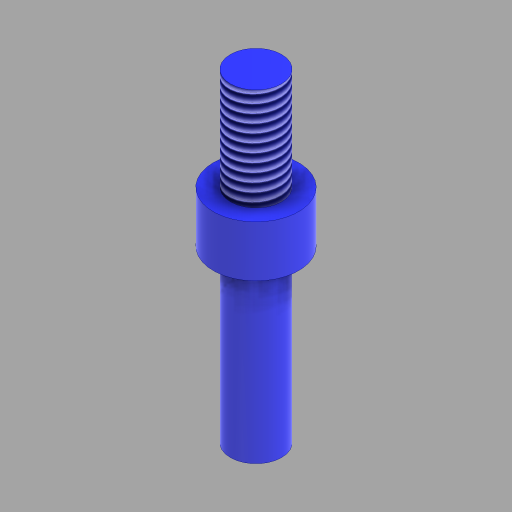
# Autodesk Inventor part: Fitting-1
Saved by Autodesk Inventor 2024 (Build 280153020, 153B)
## iProperties
Created: 2023-09-24
Part Number: Fitting-1
Material: Brass
Document SubType Name: Modeling
Designer: schanen
Density: 8.49 g/cm^3
Appearance: Blue - Wall Paint - Glossy
Author: schanen
Autodesk Inventor part; units mm, degrees
ref_plane "YZ Plane" through (0, 0, 0) normal (1, 0, 0) x (0, 1, 0)
ref_plane "XZ Plane" through (0, 0, 0) normal (0, 1, 0) x (-1, 0, 0)
ref_plane "XY Plane" through (0, 0, 0) normal (0, 0, 1) x (1, 0, 0)
sketch "Sketch1" plane through (0, 0, 0) normal (0, 0, 1) x (1, 0, 0)
  line L0 (0, 19) -> (-1.5, 19)
  line L1 (-1.5, 19) -> (-1.5, 13)
  line L2 (-1.5, 13) -> (-2.5, 13)
  line L3 (-2.5, 13) -> (-2.5, 10)
  line L4 (-2.5, 10) -> (-1.5, 10)
  line L5 (-1.5, 10) -> (-1.5, 0)
  line L6 (-1.5, 0) -> (0, 0)
  line L7 (0, 0) -> (0, 19)
  dimension "d0" = 1.5
  dimension "d1" = 1.5
  dimension "d2" = 2.5
  dimension "d3" = 10
  dimension "d4" = 6
  dimension "d5" = 3
  constraints: 16 end point, 6 perpendicular, 1 coincident, 1 horizontal, 1 vertical, 1 vertical alignment
  measures "d0" distance between parallel lines of L7 L1
  measures "d1" distance between parallel lines of L7 L5
  measures "d2" distance between parallel lines of L7 L3
  measures "d3" distance of L4.end L5.end
  measures "d4" distance of L0.end L1.end
  measures "d5" distance of L2.end L3.end
revolve "Revolution1" add sketch "Sketch1" angle 360 about axis through (0, 0, 0) along (0, 1, 0)
thread "Thread1" size "M3x0.5" class "6g" standard "ANSI Metric M Profile" full length
body "Solid1"
